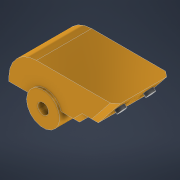
# Autodesk Inventor part: McCrea_front_walle
Saved by Autodesk Inventor 2022 (Build 260153000, 153)
## iProperties
Created: 2022-02-07
Part Number: McCrea_front_walle
Material: Generic
Document SubType Name: Modeling
Designer: student
Density: 1 g/cm^3
Appearance: Default
Author: student
Autodesk Inventor part; units mm, degrees
ref_plane "YZ Plane" through (0, 0, 0) normal (1, 0, 0) x (0, 1, 0)
ref_plane "XZ Plane" through (0, 0, 0) normal (0, 1, 0) x (-1, 0, 0)
sketch "Sketch1" plane through (0, 0, 0) normal (0, 0, 1) x (1, 0, 0)
  arc A0 (0, 125) -> (-125, 0) centre (0, 0) ccw
  line L0 (0, 125) -> (260, 125)
  line L1 (-125, 0) -> (260, 0)
  line L2 (260, 125) -> (260, 0)
  line L3 (260, 125) -> (360, 125)
  line L4 (360, 125) -> (260, 0)
  line L5 (260, 0) -> (40, 0)
  line L6 (40, 0) -> (40, -40)
  circle A1 centre (40, -40) radius 75
  circle A2 centre (40, -40) radius 25
  line L7 (40, -40) -> (175, -40)
  line L8 (175, -40) -> (215, 0)
  line L9 (40, -40) -> (-125, -40)
  line L10 (-125, -40) -> (-125, 0)
  point P0 (103.4429, 0)
  point P1 (40, 0)
  point P2 (40, -15)
  point P3 (-23.4429, 0)
  point P4 (115, -40)
  point P5 (-35, -40)
  dimension "d0" = 250
  dimension "d1" = 260
  dimension "d2" = 125
  dimension "d3" = 385
  dimension "d4" = 100
  dimension "d19" = 150
  dimension "d20" = 50
  dimension "d21" = 135
  dimension "d22" = 45
  dimension "d23" = 165
  dimension "d24" = 40
  constraints: 22 end point, 6 horizontal, 3 centre point, 2 coincident, 2 perpendicular, 2 point on circle, 1 point on line, 1 vertical
  measures "d0" diameter of A0
  measures "d1" distance of L0.start L0.end
  measures "d2" distance of L0.end L1.end
  measures "d3" distance of L1.start L1.end
  measures "d4" distance of L0.end L3.end
  measures "d19" diameter of A1
  measures "d20" diameter of A2
  measures "d21" distance of L7.start L7.end
  measures "d22" angle of L1 L8
  measures "d23" distance from line of L1.start L6
  measures "d24" distance of L5.end L6.end
extrude "Extrusion1" add sketch "Sketch1" along normal blind 250 contours L0 L2 L1 A1 A0 | L1 A1 L9 L10 | L3 L4 L2 | A1 L1 | L1 L6 A2 L9 A1 | L1 A1 L7 A2 L6 | L1 L8 L7 A1 | L9 A2 L7 A1
sketch "Sketch2" plane through (360, 125, 250) normal (0.7808688, -0.624695, 0) x (0, 0, -1)
  line L0 (250, -160.0781) -> (250, 0) projected
  line L1 (250, 0) -> (0, 0) projected
  line L2 (0, -160.0781) -> (0, 0) projected
  line L3 (250, -160.0781) -> (0, -160.0781) projected
  circle A0 centre (60, -70) radius 20
  line L4 (125, 0) -> (125, -160.0781)
  circle A1 centre (190, -70) radius 20
  point P0 (250, -322.4988)
  dimension "d7" = 60
  dimension "d8" = 70
  dimension "d9" = 40
  constraints: 2 centre point, 2 end point, 2 midpoint, 1 symmetric about line, 1 other
  measures "d7" distance from line of L2 A0.centre
  measures "d8" distance from line of L1 A0.centre
  measures "d9" diameter of A0
extrude "Extrusion2" add sketch "Sketch2" along normal blind 15 contours A0 | A1
sketch "Sketch3" plane through (0, 0, 0) normal (0, 0, -1) x (-1, 0, 0)
  point P0 (0, 0)
sketch "Sketch5" plane through (0, 0, 0) normal (0, 0, -1) x (-1, 0, 0)
  line L0 (-115, -40) -> (-175, -40) projected
  arc A0 (-115, -40) -> (35, -40) centre (-40, -40) ccw projected
  line L1 (125, -40) -> (35, -40) projected
  line L2 (125, 0) -> (125, -40) projected
  arc A1 (125, 0) -> (0, 125) centre (0, 0) ccw projected
  line L3 (-360, 125) -> (0, 125) projected
  line L4 (-260, 0) -> (-360, 125) projected
  line L5 (-215, 0) -> (-260, 0) projected
  line L6 (-175, -40) -> (-215, 0) projected
  circle A2 centre (-40, -40) radius 25 projected
  arc A3 (-115, -40) -> (35, -40) centre (-40, -40) ccw projected
  circle A4 centre (-40, -40) radius 75
  point P0 (35, -40)
  dimension "d25" = 0
  constraints: 1 centre point, 1 coincident
  measures "d25" radial gap between concentric circles of A0 A4
extrude "Extrusion4" add sketch "Sketch5" along normal blind 10 contours A4 A0
chamfer "Chamfer1" distance 20 angle 45 10 edges at (145, -40, 0) (195, -20, 0) (237.5, 0, 0) (310, 62.5, 0) (-80, -40, 0) (145, -40, 250) (195, -20, 250) (237.5, 0, 250) (310, 62.5, 250) (-80, -40, 250)
ref_plane "Work Plane1" through (0, 0, 125) normal (0, 0, -1) x (-1, 0, 0)
mirror "Mirror1" about plane through (0, 0, 125) normal (0, 0, -1) of "Extrusion4"
body "Solid1"
